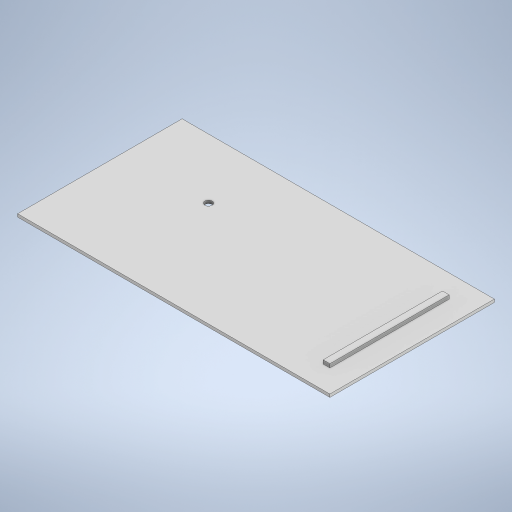
# Autodesk Inventor part: Lid
Saved by Autodesk Inventor 2023 (Build 270158000, 158)
## iProperties
Created: 2024-03-30
Part Number: Lid
Material: Generic
Document SubType Name: Modeling
Designer: lykou
Density: 1 g/cm^3
Appearance: Default
Author: lykou
Autodesk Inventor part; units mm, degrees
ref_plane "YZ Plane" through (0, 0, 0) normal (1, 0, 0) x (0, 1, 0)
ref_plane "XZ Plane" through (0, 0, 0) normal (0, 1, 0) x (-1, 0, 0)
ref_plane "XY Plane" through (0, 0, 0) normal (0, 0, 1) x (1, 0, 0)
sketch "Sketch1" plane through (0, 0, 0) normal (0, 1, 0) x (-1, 0, 0)
  line L0 (0, 0) -> (138.2, 0)
  line L1 (138.2, 0) -> (138.2, -72.8)
  line L2 (138.2, -72.8) -> (0, -72.8)
  line L3 (0, -72.8) -> (0, 0)
  dimension "d0" = 138.2
  dimension "d1" = 72.8
  constraints: 8 end point, 2 parallel, 1 horizontal, 1 perpendicular
  measures "d0" distance of L1.end L2.end
  measures "d1" distance of L0.end L1.end
extrude "Extrusion1" add sketch "Sketch1" along normal blind 1.3
sketch "Sketch2" plane through (0, 1.3, 0) normal (0, 1, 0) x (1, 0, 0)
  line L0 (0, 72.8) -> (-138.2, 72.8) projected
  line L1 (0, 72.8) -> (-100, 72.8)
  line L2 (-100, 72.8) -> (-100, 46.3)
  circle A0 centre (-100, 46.3) radius 1.65
  point P0 (0, 0)
  dimension "d4" = 100
  dimension "d5" = 26.5
  dimension "d6" = 3.3
  constraints: 4 end point, 1 centre point, 1 coincident, 1 point on line, 1 vertical
  measures "d4" distance of L0.start L1.end
  measures "d5" distance of L1.end L2.end
  measures "d6" diameter of A0
extrude "Extrusion2" cut sketch "Sketch2" against normal through all
sketch "Sketch3" plane through (0, 1.3, 0) normal (0, 1, 0) x (1, 0, 0)
  line L0 (-138.2, 0) -> (0, 0) projected
  line L1 (0, 0) -> (0, 10)
  line L2 (0, 0) -> (0, 72.8) projected
  line L3 (0, 10) -> (-10, 10)
  line L4 (0, 72.8) -> (0, 62.8)
  line L5 (0, 62.8) -> (-10, 62.8)
  line L6 (-10, 10) -> (-13, 10)
  line L7 (-13, 10) -> (-13, 62.8)
  line L8 (-13, 62.8) -> (-10, 62.8)
  line L9 (-10, 62.8) -> (-10, 10)
  dimension "d9" = 10
  dimension "d10" = 10
  dimension "d11" = 10
  dimension "d12" = 10
  dimension "d13" = 3
  constraints: 16 end point, 3 perpendicular, 3 point on line, 2 parallel, 1 horizontal
  measures "d9" distance of L0.end L1.end
  measures "d10" distance of L1.end L3.end
  measures "d11" distance of L2.end L4.end
  measures "d12" distance of L4.end L5.end
  measures "d13" distance of L7.end L8.end
extrude "Extrusion3" add sketch "Sketch3" along normal blind 1.6 contours L6 L7 L8 L9
body "Solid1"
